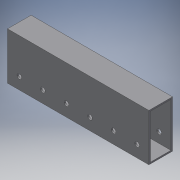
# Autodesk Inventor part: Mounting part
Saved by Autodesk Inventor 2018 (Build 220112000, 112)
## iProperties
Created: 2019-01-26
Part Number: Mounting part
Material: Generic
Document SubType Name: Modeling
Designer: s-4008082
Density: 1 g/cm^3
Appearance: Default
Author: s-4008082
Autodesk Inventor part; units mm, degrees
ref_plane "YZ Plane" through (0, 0, 0) normal (1, 0, 0) x (0, 1, 0)
ref_plane "XZ Plane" through (0, 0, 0) normal (0, 1, 0) x (-1, 0, 0)
ref_plane "XY Plane" through (0, 0, 0) normal (0, 0, 1) x (1, 0, 0)
sketch "Sketch1" plane through (0, 0, 0) normal (1, 0, 0) x (0, 1, 0)
  line L0 (-22.9273, 0) -> (27.8727, 0)
  line L1 (27.8727, 0) -> (27.8727, 25.4)
  line L2 (27.8727, 25.4) -> (-22.9273, 25.4)
  line L3 (-22.9273, 25.4) -> (-22.9273, 0)
  line L4 (26.2217, 23.749) -> (-21.2763, 23.749)
  line L5 (-21.2763, 23.749) -> (-21.2763, 1.651)
  line L6 (-21.2763, 1.651) -> (26.2217, 1.651)
  line L7 (26.2217, 1.651) -> (26.2217, 23.749)
  point P0 (0, 0)
  dimension "d0" = 25.4
  dimension "d1" = 50.8
  dimension "d2" = 1.651
  dimension "d3" = 1.651
  dimension "d4" = 1.651
  dimension "d5" = 1.651
  constraints: 16 end point, 4 parallel, 2 horizontal, 2 perpendicular
  measures "d0" distance of L0.end L1.end
  measures "d1" distance of L1.end L2.end
  measures "d2" distance between parallel lines of L2 L4
  measures "d3" distance between parallel lines of L3 L5
  measures "d4" distance between parallel lines of L0 L6
  measures "d5" distance between parallel lines of L1 L7
extrude "Extrusion1" add sketch "Sketch1" along normal blind 152.4
sketch "Sketch2" plane through (0, -22.9273, 0) normal (0, 0, -1) x (-1, 0, 0)
  circle A0 centre (-63.5, 12.7) radius 2.5797
  circle A1 centre (-88.9, 12.7) radius 2.5797
  circle A2 centre (-38.1, 12.7) radius 2.5797
  circle A3 centre (-12.7, 12.7) radius 2.5797
  circle A4 centre (-114.3, 12.7) radius 2.5797
  circle A5 centre (-139.7, 12.7) radius 2.5797
  line L0 (0, 0) -> (0, 50.8) projected
  line L1 (-152.4, 0) -> (-152.4, 50.8) projected
  line L2 (0, 0) -> (-152.4, 0) projected
  point P0 (0, 22.9273)
  dimension "d8" = 5.1594
  dimension "d9" = 5.1594
  dimension "d13" = 5.1594
  dimension "d14" = 5.1594
  dimension "d15" = 5.1594
  dimension "d16" = 5.1594
  dimension "d17" = 25.4
  dimension "d18" = 12.7
  dimension "d20" = 88.9
  dimension "d21" = 12.7
  dimension "d22" = 12.7
  dimension "d23" = 63.5
  dimension "d24" = 25.4
  dimension "d25" = 12.7
  dimension "d26" = 12.7
  dimension "d27" = 12.7
  dimension "d28" = 12.7
  dimension "d29" = 12.7
  constraints: 6 centre point
  measures "d8" diameter of A5
  measures "d9" diameter of A4
  measures "d13" diameter of A0
  measures "d14" diameter of A1
  measures "d15" diameter of A2
  measures "d16" diameter of A3
  measures "d17" distance of A2.centre A3.centre
  measures "d18" distance from line of L0 A3.centre
  measures "d20" distance from line of L1 A0.centre
  measures "d21" distance from line of L2 A1.centre
  measures "d22" distance from line of L2 A0.centre
  measures "d23" distance from line of L1 A1.centre
  measures "d24" distance of A4.centre A5.centre
  measures "d25" distance from line of L1 A5.centre
  measures "d26" distance from line of L2 A5.centre
  measures "d27" distance from line of L2 A4.centre
  measures "d28" distance from line of L2 A2.centre
  measures "d29" distance from line of L2 A3.centre
extrude "Extrusion2" cut sketch "Sketch2" against normal blind 25.4
equation "\"d3\" = d2"
equation "\"d4\" = d2"
equation "\"d5\" = d2"
equation "\"d9\" = d8"
equation "\"d13\" = d8"
equation "\"d14\" = d8"
equation "\"d15\" = d8"
equation "\"d16\" = d8"
equation "\"d22\" = d21"
equation "\"d26\" = d21"
equation "\"d27\" = d21"
equation "\"d28\" = d21"
equation "\"d29\" = d21"
body "Solid1"
